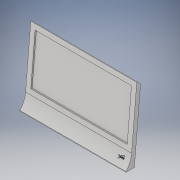
# Autodesk Inventor part: terminal use
Saved by Autodesk Inventor 2017 (Build 210142000, 142)
## iProperties
Created: 2018-03-12
Part Number: terminal use
Material: Generic
Document SubType Name: Modeling
Designer: Braxton
Density: 1 g/cm^3
Appearance: Default
Author: Braxton
Autodesk Inventor part; units mm, degrees
ref_plane "YZ Plane" through (0, 0, 0) normal (1, 0, 0) x (0, 1, 0)
ref_plane "XZ Plane" through (0, 0, 0) normal (0, 1, 0) x (-1, 0, 0)
ref_plane "XY Plane" through (0, 0, 0) normal (0, 0, 1) x (1, 0, 0)
sketch "Sketch1" plane through (0, 0, 0) normal (0, 0, 1) x (1, 0, 0)
  line L0 (0, 0) -> (0, 29.8979)
  line L1 (0, 29.8979) -> (43.6562, 29.8979)
  line L2 (43.6562, 29.8979) -> (43.6562, 0)
  line L3 (43.6562, 0) -> (0, 0)
  dimension "d0" = 29.8979
  dimension "d1" = 43.6562
  constraints: 8 end point, 3 perpendicular, 1 horizontal
  measures "d0" distance of L0.start L0.end
  measures "d1" distance of L0.end L1.end
extrude "block to cut from" add sketch "Sketch1" along normal blind 14.0396
sketch "Sketch2" plane through (43.6562, 0, 0) normal (1, 0, 0) x (0, 0, -1)
  line L0 (0, 0) -> (0, 29.8979) projected
  line L1 (0, 0) -> (0, 0.2646)
  line L2 (0, 0.2646) -> (-7.9375, 0.2646)
  line L3 (-7.9375, 0.2646) -> (-6.404, 17.7924)
  line L4 (-14.0396, 29.8979) -> (-14.0396, 0) projected
  line L5 (0, 0) -> (-14.0396, 0) projected
  line L6 (0, 29.8979) -> (-14.0396, 29.8979) projected
  line L7 (-9.5879, 29.8979) -> (-9.3233, 29.8979)
  line L8 (-9.3233, 29.8979) -> (-8.1073, 28.6818)
  line L9 (-8.1073, 28.6818) -> (-10.5934, 0.2646) construction
  line L10 (-9.5879, 29.8979) -> (-11.7094, 5.6489)
  arc A0 (-14.0397, 0.2646) -> (-11.7094, 5.6489) centre (-20.9665, 6.4588) ccw
  line L11 (-14.0397, 0.2646) -> (-10.5934, 0.2646)
  line L12 (-10.5934, 0.2646) -> (-7.9375, 0.2646)
  arc A1 (-7.6347, 20.5424) -> (-6.404, 17.7924) centre (-3.0629, 20.938) ccw
  arc A2 (-8.1073, 28.6818) -> (-7.6347, 20.5424) centre (135.7265, 32.9486) ccw
  line L13 (-14.0397, 0.2646) -> (-14.0396, 29.8979)
  line L14 (-14.0396, 29.8979) -> (-9.5879, 29.8979)
  line L15 (-9.3233, 29.8979) -> (0, 29.8979)
  line L16 (0, 29.8979) -> (0, 0.2646)
  dimension "d4" = 0.2646
  dimension "d6" = 7.9375
  dimension "d7" = 85
  dimension "d8" = 17.5948
  dimension "d12" = 0.2646
  dimension "d13" = 1.7198
  dimension "d14" = 135
  dimension "d15" = 2.6458
  dimension "d16" = 24.3417
  dimension "d17" = 1.8521
  dimension "d19" = 4.5889
  dimension "d20" = 143.897
  constraints: 26 end point, 6 point on circle, 4 collinear, 3 centre point, 3 point on line, 2 parallel, 2 tangent, 1 horizontal, 1 perpendicular
  measures "d4" distance of L0.start L1.end
  measures "d6" distance of L1.end L2.end
  measures "d7" angle of L3 L2
  measures "d8" distance of L2.end L3.end
  measures "d12" distance of L7.start L7.end
  measures "d13" distance of L7.end L8.end
  measures "d14" angle of L6 L8
  measures "d15" distance between parallel lines of L3 L9
  measures "d16" distance of L7.start L10.end
  measures "d17" distance from line of L11.start L10
  measures "d19" radius of A1
  measures "d20" radius of A2
extrude "side view correct" cut sketch "Sketch2" against normal up to next contours L2 L3 A1 A2 L8 L6 L0 | L4 L6 L10 A0
sketch "Sketch3" plane through (43.6562, 0.2646, 7.9375) normal (0, 1, 0) x (1, 0, 0)
  line L0 (0, 0) -> (0, 1.5335) projected
  line L1 (0, 0) -> (-8.4667, 0)
  line L2 (0, 0) -> (-43.6562, 0) projected
  line L3 (-43.6562, 1.5335) -> (-43.6562, 0) projected
  line L4 (-43.6562, 0) -> (-35.1896, 0)
  line L5 (-43.6562, 7.9375) -> (-43.6562, -6.1021) projected
  line L6 (-43.6562, 0) -> (-43.6562, 7.9375)
  line L7 (-43.6562, 7.9375) -> (-21.8281, 7.9375)
  line L8 (-21.8281, 7.9375) -> (0, 7.9375)
  line L9 (0, 7.9375) -> (0, 0)
  arc A0 (-8.4667, 0) -> (-35.1896, 0) centre (-21.8281, -7.2771) ccw
  dimension "d23" = 8.4667
  dimension "d24" = 8.4667
  constraints: 12 end point, 3 point on circle, 2 point on line, 1 centre point, 1 collinear, 1 perpendicular
  measures "d23" distance of L0.start L1.end
  measures "d24" distance of L2.end L4.end
extrude "top view correct" cut sketch "Sketch3" against normal up to next contours L1 A0 L8 L9 L0 | L2 L3 L5 L7 A0
ref_plane "Work Plane1" through (43.6562, 17.7924, 6.404) normal (0, -0.9961947, 0.0871557) x (-1, 0, 0)
sketch "Sketch4" plane through (43.6562, 17.7924, 6.404) normal (0, -0.9961947, 0.0871557) x (-1, 0, 0)
  ellipse E0 centre (21.8281, -7.2495) end of major axis (6.6135, -7.2495) minor radius 15.1567 (35.1896, 0) -> (8.4667, 0) ccw projected
  line L0 (0, -2.6458) -> (0, -1.4657) projected
  line L1 (1.1225, -1.4657) -> (1.5875, -1.4657)
  arc A0 (7.3492, -0.8384) -> (8.4667, 0) centre (6.9861, 0.8094) ccw
  arc A1 (1.5875, -1.4657) -> (7.3492, -0.8384) centre (1.5875, 25.3083) ccw
  line L2 (21.8281, -7.7992) -> (21.8281, 9.6278)
  line L3 (0, 0.0231) -> (0, -6.0559) projected
  line L4 (0, -1.4657) -> (0, 0.0231)
  line L5 (43.6562, -1.4657) -> (0, -1.4657) construction
  line L6 (42.5337, -1.4657) -> (42.0687, -1.4657)
  arc A2 (35.1896, 0) -> (36.307, -0.8384) centre (36.6701, 0.8094) ccw
  arc A3 (36.307, -0.8384) -> (42.0687, -1.4657) centre (42.0687, 25.3083) ccw
  line L7 (43.6562, -1.4657) -> (43.6562, 0.0231)
  line L8 (8.4667, 0) -> (8.4667, 0.0231) projected
  line L9 (8.4667, 0) -> (8.4667, 0.0231)
  line L10 (8.4667, 0.0231) -> (0, 0.0231) projected
  line L11 (8.4667, 0.0231) -> (0, 0.0231)
  line L12 (43.6562, 0.0231) -> (35.1896, 0.0231) projected
  line L13 (35.1896, 0) -> (35.1896, 0.0231) projected
  line L14 (35.1896, 0.0231) -> (35.1896, 0)
  line L15 (35.1896, 0) -> (35.1896, 0.0231)
  ellipse E1 centre (21.8281, -7.2264) end of major axis (37.0428, -7.2264) minor radius 15.1567 (35.1896, 0.0231) -> (8.4667, 0.0231) ccw projected
  line L16 (43.6562, 0.0231) -> (35.1896, 0.0231)
  line L17 (0, -2.5882) -> (1.1225, -1.4657)
  line L18 (43.6562, -2.5882) -> (42.5337, -1.4657)
  line L19 (0, -1.4657) -> (0, -2.5882)
  line L20 (43.6562, -1.4657) -> (43.6562, -2.5882)
  line L21 (43.6562, 0.0231) -> (43.6562, -6.0559) projected
  point P0 (43.6562, 7.9304)
  dimension "d28" = 1.5875
  dimension "d38" = 1.5875
  dimension "d40" = 45
  constraints: 30 end point, 8 point on circle, 7 symmetric about line, 5 collinear, 4 centre point, 2 horizontal, 2 point on line, 2 vertical, 1 perpendicular, 1 tangent, 5 other
  measures "d28" distance of L0.end L1.end
  measures "d38" distance of L1.start L17.start
  measures "d40" angle of L17 L0
extrude "slight top view correction" cut sketch "Sketch4" along normal mid plane 37.8354 contours L13 L12 L7 L20 L18 L6 A3 A2 | A0 A1 L1 L17 L0 L3 L10 L8
sketch "Sketch5" plane through (0, 5.6489, 11.7094) normal (0, 0.0871557, 0.9961947) x (1, 0, 0)
  line L0 (0, 0) -> (0, 24.3417) projected
  line L1 (0, 12.1708) -> (1.9844, 12.1708)
  line L2 (0, 24.3417) -> (43.6562, 24.3417) projected
  line L3 (21.8281, 24.3417) -> (21.8281, 22.225)
  line L4 (43.6562, 24.3417) -> (43.6562, 0) projected
  line L5 (43.6562, 12.1708) -> (41.6719, 12.1708)
  line L6 (43.6562, 0) -> (0, 0) projected
  line L7 (21.8281, 0) -> (21.8281, 2.1167)
  line L8 (1.9844, 22.225) -> (41.6719, 22.225)
  line L9 (41.6719, 22.225) -> (41.6719, 2.1167)
  line L10 (41.6719, 2.1167) -> (1.9844, 2.1167)
  line L11 (1.9844, 2.1167) -> (1.9844, 22.225)
  point P0 (0, -4.6068)
  dimension "d32" = 1.9844
  dimension "d33" = 2.1167
  dimension "d34" = 1.9844
  dimension "d35" = 2.1167
  constraints: 16 end point, 8 midpoint, 2 horizontal, 2 parallel, 2 perpendicular, 2 vertical
  measures "d32" distance of L1.start L1.end
  measures "d33" distance of L3.start L3.end
  measures "d34" distance of L5.start L5.end
  measures "d35" distance of L7.start L7.end
extrude "screen" cut sketch "Sketch5" against normal blind 0.5292 contours L11 L8 L9 L10
ref_plane "Work Plane2" through (43.6562, 0.2646, 14.0396) normal (0, -0.3971809, -0.9177403) x (-1, 0, 0)
sketch "Sketch7" plane through (43.6562, 0.2646, 14.0396) normal (0, -0.3971809, -0.9177403) x (-1, 0, 0)
  line L0 (0, 0) -> (0, 5.8669) projected
  line L1 (0, 2.9335) -> (2.3823, 2.9335)
  line L2 (2.3823, 2.6668) -> (2.3823, 3.2002)
  line L3 (2.3823, 3.2002) -> (4.3169, 3.2002)
  line L4 (2.3823, 2.6668) -> (4.3169, 2.6668)
  line L5 (4.3169, 2.6668) -> (4.3169, 3.2002)
  point P0 (43.6562, 5.3335)
  dimension "d49" = 2.3823
  dimension "d50" = 1.9346
  dimension "d51" = 0.5334
  constraints: 10 end point, 3 horizontal, 2 midpoint, 1 perpendicular, 1 vertical
  measures "d49" distance of L1.start L1.end
  measures "d50" distance of L2.end L3.end
  measures "d51" distance of L2.start L2.end
extrude "light cutout" cut sketch "Sketch7" along normal blind 0.762
sketch "Sketch8" plane through (43.6562, -0.0381, 13.3403) normal (0, 0.3971809, 0.9177403) x (1, 0, 0)
  line L0 (-4.3011, 3.1684) -> (-2.3982, 3.1684)
  line L1 (-4.3169, 3.2002) -> (-2.3823, 3.2002) projected
  line L2 (-2.3982, 3.1684) -> (-2.3982, 2.6985)
  line L3 (-2.3823, 3.2002) -> (-2.3823, 2.6668) projected
  line L4 (-4.3011, 3.1684) -> (-4.3011, 2.6985)
  line L5 (-4.3011, 2.6985) -> (-2.3982, 2.6985)
  line L6 (-2.3823, 2.6668) -> (-4.3169, 2.6668) projected
  line L7 (-2.83, 3.1684) -> (-2.83, 2.6985)
  point P0 (-43.6562, 5.3335)
  point P1 (-3.3496, 3.1684)
  point P2 (-3.3496, 3.2002)
  point P3 (-2.3982, 2.9335)
  point P4 (-2.3823, 2.9335)
  dimension "d54" = 1.9029
  dimension "d55" = 0.0318
  dimension "d56" = 0.4699
  dimension "d59" = 0.4318
  constraints: 10 end point, 4 midpoint, 2 point on line, 2 vertical, 1 horizontal, 1 parallel, 1 perpendicular
  measures "d54" distance of L0.start L0.end
  measures "d55" distance between parallel lines of L1 L0
  measures "d56" distance of L0.end L2.end
  measures "d59" distance between parallel lines of L2 L7
extrude "power indicator" add sketch "Sketch8" along normal up to surface separate body contours L0 L2 L5 L7 round surface about axis through (43.6562, 6.4588, 20.9665) along (-1, 0, 0) radius 9.2924 far side no
extrude "power button" add sketch "Sketch8" along normal blind 0.347 separate body contours L0 L7 L5 L4
sketch "Sketch11" plane through (43.6562, 0.0998, 13.6588) normal (0, 0.3971809, 0.9177403) x (1, 0, 0)
  line L0 (-2.83, 3.1684) -> (-4.3011, 3.1684) projected
  line L1 (-4.3011, 3.1684) -> (-2.83, 3.1684)
  line L2 (-2.83, 3.1684) -> (-2.83, 2.6985) projected
  line L3 (-2.83, 3.1684) -> (-2.83, 2.6985)
  line L4 (-3.5655, 3.1684) -> (-3.5655, 2.9622) construction
  line L5 (-3.5655, 2.9335) -> (-2.83, 2.9335) construction
  arc A0 (-3.6098, 3.0637) -> (-3.6176, 3.0868) centre (-3.6137, 3.0752) ccw
  line L6 (-3.5655, 2.9335) -> (-3.5655, 3.1306) construction
  arc A1 (-3.5135, 3.0868) -> (-3.5213, 3.0637) centre (-3.5174, 3.0752) ccw
  arc A2 (-3.6176, 3.0868) -> (-3.5135, 3.0868) centre (-3.5655, 2.9335) ccw
  arc A3 (-3.6098, 3.0637) -> (-3.5213, 3.0637) centre (-3.5655, 2.9335) ccw
  point P0 (-43.6562, 5.3335)
  point P1 (-3.5655, 3.032)
  dimension "d73" = 0.0481
  constraints: 11 end point, 8 point on circle, 4 centre point, 3 midpoint, 3 symmetric about line, 2 collinear, 2 point on line, 1 horizontal, 1 vertical, 1 other
  measures "d73" distance from line of L4 A0.centre
equation "\"d24\" = d23"
equation "\"d34\" = d32"
equation "\"d35\" = d33"
body "Solid1"
body "Solid2"
body "Solid3"
